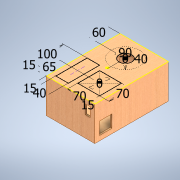
# Autodesk Inventor part: estruc_mec
Saved by Autodesk Inventor 2022 (Build 260153000, 153)
## iProperties
Created: 2022-03-21
Part Number: estruc_mec
Material: Wood (Cherry)
Document SubType Name: Modeling
Designer: User
Density: 0.63 g/cm^3
Appearance: Cherry - Natural Low Gloss
Author: User
Autodesk Inventor part; units mm, degrees
ref_plane "YZ Plane" through (0, 0, 0) normal (1, 0, 0) x (0, 1, 0)
ref_plane "XZ Plane" through (0, 0, 0) normal (0, 1, 0) x (-1, 0, 0)
ref_plane "XY Plane" through (0, 0, 0) normal (0, 0, 1) x (1, 0, 0)
sketch "Sketch1" plane through (0, 0, 0) normal (0, 1, 0) x (-1, 0, 0)
  line L0 (-77.5, 117.5) -> (77.5, 117.5)
  line L1 (77.5, 117.5) -> (77.5, -117.5)
  line L2 (77.5, -117.5) -> (-77.5, -117.5)
  line L3 (-77.5, -117.5) -> (-77.5, 117.5)
  line L4 (-77.5, 117.5) -> (77.5, -117.5) construction
  line L5 (77.5, 117.5) -> (-77.5, -117.5) construction
  point P0 (0, 0)
  dimension "d0" = 235
  dimension "d1" = 155
  constraints: 12 end point, 2 midpoint, 2 parallel, 1 horizontal, 1 perpendicular
  measures "d0" distance of L0.end L1.end
  measures "d1" distance of L0.start L0.end
extrude "Extrusion1" add sketch "Sketch1" along normal mid plane 110
shell "Shell1" thickness 5 removed faces 1 at (25.8333, 55, 39.1667)
sketch "Sketch2" plane through (-72.5, -50, -112.5) normal (0, 0, 1) x (1, 0, 0)
  line L0 (0, 0) -> (0, 105) projected
  line L1 (145, 105) -> (145, 0) projected
  line L2 (0, 105) -> (145, 105)
  line L3 (145, 105) -> (145, 100)
  line L4 (145, 100) -> (0, 100)
  line L5 (0, 100) -> (0, 105)
  point P0 (72.5, 50)
  point P1 (145, 105)
  dimension "d5" = 5
  constraints: 8 end point, 2 parallel, 1 horizontal, 1 perpendicular, 1 point on line
  measures "d5" distance of L3.end L1.start
extrude "Extrusion2" add sketch "Sketch2" along normal through all
sketch "Sketch3" plane through (0, 55, 0) normal (0, 1, 0) x (1, 0, 0)
  line L0 (62.5, -87.5) -> (-7.5, -87.5)
  line L1 (-7.5, -87.5) -> (-7.5, -17.5)
  line L2 (-7.5, -17.5) -> (62.5, -17.5)
  line L3 (62.5, -17.5) -> (62.5, -87.5)
  line L4 (62.5, -87.5) -> (-7.5, -17.5) construction
  line L5 (-7.5, -87.5) -> (62.5, -17.5) construction
  line L6 (-77.5, 117.5) -> (-77.5, -117.5) projected
  line L7 (-77.5, -117.5) -> (77.5, -117.5) projected
  line L8 (77.5, 117.5) -> (-77.5, 117.5) projected
  circle A0 centre (0, 57.5) radius 20
  line L9 (77.5, -117.5) -> (77.5, 117.5) projected
  line L10 (-62.5, -102.5) -> (-22.5, -102.5)
  line L11 (-22.5, -102.5) -> (-22.5, -2.5)
  line L12 (-22.5, -2.5) -> (-62.5, -2.5)
  line L13 (-62.5, -2.5) -> (-62.5, -102.5)
  circle A1 centre (0, 57.5) radius 45 construction
  point P0 (0, 0)
  point P1 (27.5, -52.5)
  point P2 (-42.5, -52.5)
  dimension "d12" = 70
  dimension "d13" = 70
  dimension "d20" = 40
  dimension "d31" = 15
  dimension "d32" = 100
  dimension "d33" = 40
  dimension "d34" = 15
  dimension "d35" = 15
  dimension "d37" = 0
  dimension "d38" = 65
  dimension "d40" = 0
  dimension "d41" = 60
  dimension "d42" = 90
  constraints: 20 end point, 4 parallel, 2 centre point, 2 horizontal, 2 midpoint, 2 perpendicular, 1 coincident
  measures "d12" distance of L1.end L2.end
  measures "d13" distance of L2.end L0.start
  measures "d20" diameter of A0
  measures "d31" distance between parallel lines of L9 L3
  measures "d32" distance of L12.end L10.start
  measures "d33" distance of L11.end L12.end
  measures "d34" distance between parallel lines of L6 L13
  measures "d35" distance between parallel lines of L7 L10
  measures "d37" vertical distance of point (27.5, -52.5) point (-42.5, -52.5)
  measures "d38" distance from line of L7 point (-42.5, -52.5)
  measures "d40" horizontal distance of point (0, 0) A0.centre
  measures "d41" distance from line of L8 A0.centre
  measures "d42" diameter of A1
sketch "Sketch4" plane through (77.5, -55, -117.5) normal (1, 0, 0) x (0, 0, -1)
  line L0 (-220, 55) -> (-180, 55)
  line L1 (-180, 55) -> (-180, 15)
  line L2 (-180, 15) -> (-220, 15)
  line L3 (-220, 15) -> (-220, 55)
  line L4 (0, 0) -> (-235, 0) projected
  line L5 (-235, 0) -> (-235, 110) projected
  point P0 (-117.5, 55)
  dimension "d23" = 40
  dimension "d24" = 40
  dimension "d25" = 15
  dimension "d26" = 15
  constraints: 8 end point, 2 parallel, 1 horizontal, 1 perpendicular
  measures "d23" distance of L0.start L0.end
  measures "d24" distance of L2.end L0.start
  measures "d25" distance between parallel lines of L4 L2
  measures "d26" distance between parallel lines of L5 L3
sketch "Sketch5" plane through (-77.5, 55, 117.5) normal (0, 0, 1) x (1, 0, 0)
  line L0 (125, -15) -> (140, -15)
  line L1 (140, -15) -> (140, -45)
  line L2 (140, -45) -> (125, -45)
  line L3 (125, -45) -> (125, -15)
  line L4 (0, 0) -> (155, 0) projected
  line L5 (155, -110) -> (155, 0) projected
  point P0 (77.5, -55)
  dimension "d27" = 30
  dimension "d28" = 15
  dimension "d29" = 15
  dimension "d30" = 15
  constraints: 8 end point, 2 parallel, 1 horizontal, 1 perpendicular
  measures "d27" distance of L2.end L0.start
  measures "d28" distance of L1.end L2.end
  measures "d29" distance between parallel lines of L0 L4
  measures "d30" distance between parallel lines of L5 L1
sketch "Sketch6" plane through (-72.5, -50, -112.5) normal (0, 1, 0) x (1, 0, 0)
  line L0 (0, 0) -> (145, 0) construction
  line L1 (-5, -230) -> (-5, 5) construction
  line L2 (0, 0) -> (0, -100) construction
  line L3 (0, -225) -> (0, 0) projected
  line L4 (145, 0) -> (145, -225) projected
  line L5 (0, -100) -> (145, -100)
  line L6 (145, -100) -> (145, -105) construction
  line L7 (145, -105) -> (0, -105)
  line L8 (0, -105) -> (0, -100) construction
  line L9 (0, -100) -> (0, -105)
  line L10 (145, -100) -> (145, -105)
  point P0 (72.5, -112.5)
  point P1 (0, -105)
  dimension "d44" = 100
  dimension "d45" = 5
  constraints: 14 end point, 2 parallel, 2 perpendicular, 2 point on line, 1 collinear, 1 horizontal
  measures "d44" distance of L0.start L2.end
  measures "d45" distance between parallel lines of L7 L5
extrude "Extrusion3" add sketch "Sketch6" along normal through all
extrude "Extrusion4" cut sketch "Sketch3" against normal blind 10 contours A0
extrude "Extrusion5" cut sketch "Sketch4" against normal blind 10
extrude "Extrusion6" cut sketch "Sketch5" against normal blind 10
extrude "Extrusion7" cut sketch "Sketch3" against normal blind 0.1 contours L0 L1 L2 L3 | L13 L12 L11 L10
body "Solid1"
